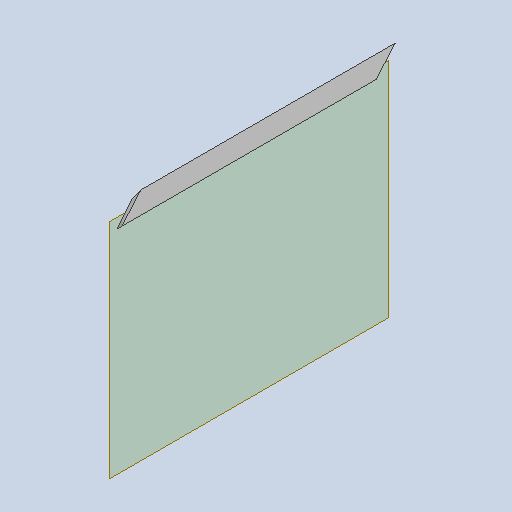
# Autodesk Inventor part: nóż
Saved by Autodesk Inventor 2022 (Build 260153000, 153)
## iProperties
Created: 2022-12-09
Part Number: nóż
Material: Generic
Document SubType Name: Modeling
Designer: Kamil
Density: 1 g/cm^3
Appearance: Default
Author: Kamil
Autodesk Inventor part; units mm, degrees
ref_plane "YZ Plane" through (0, 0, 0) normal (1, 0, 0) x (0, 1, 0)
ref_plane "XZ Plane" through (0, 0, 0) normal (0, 1, 0) x (-1, 0, 0)
ref_plane "XY Plane" through (0, 0, 0) normal (0, 0, 1) x (1, 0, 0)
sketch "Sketch1" plane through (0, 0, 0) normal (0, 0, 1) x (1, 0, 0)
  line L0 (0, 57.4166) -> (-5, 46.6664) projected
  line L1 (-5, 42.7444) -> (-5, 46.6664) projected
  line L2 (-5, 42.7444) -> (-29.7, 18.0444) projected
  line L3 (-29.7, 18.0444) -> (-29.7, -5.3095) projected
  arc A0 (-5, 0) -> (-29.7, -5.3095) centre (-13.6, -20.1) ccw projected
  line L4 (0, 0) -> (-5, 0) projected
  line L5 (0, 0) -> (0, 57.4166) projected
  circle A1 centre (-13.6, -20.1) radius 16.1 projected
  line L6 (2.5, -20.1) -> (2.5, 68.8205)
  line L7 (-13.6, -36.2) -> (-13.6, 63.8)
  line L8 (-13.6, 63.8) -> (7.5508, 63.8)
  line L9 (-5, 46.6664) -> (2.5, 62.7917)
  line L10 (2.5, 62.7917) -> (-1.25, 57.4166)
  line L11 (-1.25, 57.4166) -> (-6.961, 44.7054)
  line L12 (-6.961, 44.7054) -> (-5, 46.6664)
  dimension "d0" = 100
  constraints: 14 end point, 2 point on circle, 2 point on line, 2 vertical, 1 horizontal, 1 tangent
  measures "d0" distance of L7.start L7.end
extrude "Extrusion1" add sketch "Sketch1" against normal blind 100 contours L0 L12 L11 L10 L9
ref_plane "Work Plane1" through (-5, 15.8, -50) normal (-1, 0, 0) x (0, 0, 1)
body "Solid1"
